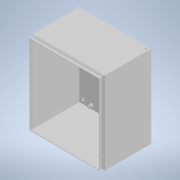
# Autodesk Inventor part: F161410HC1
Saved by Autodesk Inventor 2021 (Build 250183000, 183)
## iProperties
Created: 2025-08-10
Part Number: F161410HC1
Material: Generic
Catalog Web Link: www.cadenas.de
Description: JB CS Frame-JB
Vendor: RITTAL
Document SubType Name: Modeling
Designer: psAdmin
Manufacturer: RITTAL
Mass: 768.935 g
Surface Area: 10280.7 cm^2
Volume: 768.935 cm^3
Density: 1 g/cm^3
Appearance: PSOLRGB-175-175-175
Category: PARTsolutions
Company: RITTAL
Title: F161410HC1
Author: Cadenas PARTsolutions
Comments: JB
PSOL_IDENT_0: {$CADENAS_DATA/23d-libs/rittal/schaltschranksys/kleingeh/jb_parts/jb_frame.prj},178 {VTYP=3D},{NB=F1
PSOL_IDENT_1: 61410HC1},{LINA=F161410HC1},{NN=JB CS Frame},{DATE=20.08.2024 09:27:20},{GEOMDATE=07.07.2022 12:44:2
PSOL_IDENT_2: 1},{VERSION=},{LINEID=220},{WBVAR=DETAIL},{WBNUMERIC=DETAIL}  {NB=F161410HC1},{LINA=F161410HC1},{KT=
PSOL_IDENT_3: DUMMY},{PN=161410HC},{PNPLATE=JBMP1614},{WT=1.5000},{DETAIL=1},{WN=Y},{HM=400.00000},{BM=350.00000},
PSOL_IDENT_4: {TM=250.00000},{ST=224.03000},{ETFT=8.19000},{EPD=21.13000},{HHD=311.00000},{VHD=361.00000},{DMHD=28
PSOL_IDENT_5: 4.40000},{EW=0.00000},{EH=0.00000},{MPX=225.00000},{MPY=361.00000},{MPN=4},{NOH=2},{MAT=CS},{MT=cs}
NB: F161410HC1
NN: JB CS Frame
NT: JB
NBSYN: F$PN.$DETAIL.
LINA: F161410HC1
CATALOG: Rittal
PN: 161410HC
PNPLATE: JBMP1614
WT: 1.5
DETAIL: High
WN: Y
HM: 400
BM: 350
TM: 250
ST: 224.03
ETFT: 8.19
EPD: 21.13
HHD: 311
VHD: 361
DMHD: 284.4
EW: 0
EH: 0
MPX: 225
MPY: 361
MPN: 4
NOH: 2
MAT: CS
MT: cs
SUPPLIER: RITTAL
ARTICLENO: F161410HC1
BOMINFO: F161410HC1
CREATOR: CADENAS GmbH
Autodesk Inventor part; units mm, degrees
sketch "Sketch_1" plane through (0, 0, 0) normal (0, 0, 1) x (-1, 0, 0)
  line L0 (-175, -200) -> (175, -200)
  line L1 (175, -200) -> (175, 200)
  line L2 (175, 200) -> (-175, 200)
  line L3 (-175, 200) -> (-175, -200)
  constraints: 8 end point
extrude "Extrusion1" add sketch "Sketch_1" along normal blind 225.65
sketch "Sketch_2" plane through (0, 0, 1.5) normal (0, 0, 1) x (-1, 0, 0)
  line L0 (-173.5, -198.5) -> (173.5, -198.5)
  line L1 (173.5, -198.5) -> (173.5, 198.5)
  line L2 (173.5, 198.5) -> (-173.5, 198.5)
  line L3 (-173.5, 198.5) -> (-173.5, -198.5)
  constraints: 8 end point
extrude "Extrusion2" cut sketch "Sketch_2" along normal blind 225.65
sketch "Sketch_3" plane through (0, 0, 0) normal (-1, 0, 0) x (0, 0, -1)
  line L0 (-246.59, -193.8538) -> (-238.9625, -191.81)
  line L1 (-238.9625, -191.81) -> (-234.2713, -191.81)
  line L2 (-234.2713, -191.81) -> (-226.3742, -199.7071)
  arc A0 (-226.3742, -199.7071) -> (-225.6671, -200) centre (-225.6671, -199) ccw
  line L3 (-225.6671, -200) -> (-225.46, -200)
  line L4 (-225.46, -200) -> (-225.46, -198.5)
  line L5 (-225.46, -198.5) -> (-233.65, -190.31)
  line L6 (-233.65, -190.31) -> (-239.16, -190.31)
  line L7 (-239.16, -190.31) -> (-246.59, -192.3009)
  line L8 (-246.59, -192.3009) -> (-246.59, -193.8538)
  constraints: 18 end point, 2 point on circle, 1 centre point
extrude "Extrusion3" add sketch "Sketch_3" along normal mid plane 350
sketch "Sketch_4" plane through (0, 0, 0) normal (-1, 0, 0) x (0, 0, -1)
  line L0 (-246.59, 193.8538) -> (-246.59, 192.3009)
  line L1 (-246.59, 192.3009) -> (-239.16, 190.31)
  line L2 (-239.16, 190.31) -> (-233.65, 190.31)
  line L3 (-233.65, 190.31) -> (-225.46, 198.5)
  line L4 (-225.46, 198.5) -> (-225.46, 200)
  line L5 (-225.46, 200) -> (-225.6671, 200)
  arc A0 (-225.6671, 200) -> (-226.3742, 199.7071) centre (-225.6671, 199) ccw
  line L6 (-226.3742, 199.7071) -> (-234.2713, 191.81)
  line L7 (-234.2713, 191.81) -> (-238.9625, 191.81)
  line L8 (-238.9625, 191.81) -> (-246.59, 193.8538)
  constraints: 18 end point, 2 point on circle, 1 centre point
extrude "Extrusion4" add sketch "Sketch_4" along normal mid plane 350
sketch "Sketch_5" plane through (0, 0, 0) normal (0, -1, 0) x (-1, 0, 0)
  line L0 (-175, -225.65) -> (-166.81, -233.84)
  line L1 (-166.81, -233.84) -> (-166.81, -238.3425)
  line L2 (-166.81, -238.3425) -> (-169.0708, -246.78)
  line L3 (-169.0708, -246.78) -> (-167.5179, -246.78)
  line L4 (-167.5179, -246.78) -> (-165.31, -238.54)
  line L5 (-165.31, -238.54) -> (-165.31, -233.84)
  line L6 (-165.31, -233.84) -> (-173.5, -225.65)
  line L7 (-173.5, -225.65) -> (-175, -225.65)
  constraints: 16 end point
extrude "Extrusion5" add sketch "Sketch_5" along normal mid plane 400
sketch "Sketch_6" plane through (0, 0, 0) normal (0, -1, 0) x (-1, 0, 0)
  line L0 (165.31, -238.54) -> (167.5179, -246.78)
  line L1 (167.5179, -246.78) -> (169.0708, -246.78)
  line L2 (169.0708, -246.78) -> (166.81, -238.3425)
  line L3 (166.81, -238.3425) -> (166.81, -233.84)
  line L4 (166.81, -233.84) -> (175, -225.65)
  line L5 (175, -225.65) -> (173.5, -225.65)
  line L6 (173.5, -225.65) -> (165.31, -233.84)
  line L7 (165.31, -233.84) -> (165.31, -238.54)
  constraints: 16 end point
extrude "Extrusion6" add sketch "Sketch_6" along normal mid plane 400
sketch "Sketch_7" plane through (155, 0, 0) normal (-1, 0, 0) x (0, 0, -1)
  arc A0 (-3.5, -187.5) -> (-2, -189) centre (-2, -187.5) ccw
  line L0 (-2, -189) -> (0, -189)
  line L1 (0, -189) -> (0, -171)
  line L2 (0, -171) -> (-2, -171)
  arc A1 (-2, -171) -> (-3.5, -172.5) centre (-2, -172.5) ccw
  line L3 (-3.5, -172.5) -> (-3.5, -187.5)
  constraints: 8 end point, 4 point on circle, 2 centre point
extrude "Extrusion7" add sketch "Sketch_7" along normal mid plane 18
sketch "Sketch_8" plane through (-155, 0, 0) normal (-1, 0, 0) x (0, 0, -1)
  arc A0 (-3.5, -187.5) -> (-2, -189) centre (-2, -187.5) ccw
  line L0 (-2, -189) -> (0, -189)
  line L1 (0, -189) -> (0, -171)
  line L2 (0, -171) -> (-2, -171)
  arc A1 (-2, -171) -> (-3.5, -172.5) centre (-2, -172.5) ccw
  line L3 (-3.5, -172.5) -> (-3.5, -187.5)
  constraints: 8 end point, 4 point on circle, 2 centre point
extrude "Extrusion8" add sketch "Sketch_8" along normal mid plane 18
sketch "Sketch_9" plane through (155, 0, 0) normal (-1, 0, 0) x (0, 0, -1)
  arc A0 (-3.5, 172.5) -> (-2, 171) centre (-2, 172.5) ccw
  line L0 (-2, 171) -> (0, 171)
  line L1 (0, 171) -> (0, 189)
  line L2 (0, 189) -> (-2, 189)
  arc A1 (-2, 189) -> (-3.5, 187.5) centre (-2, 187.5) ccw
  line L3 (-3.5, 187.5) -> (-3.5, 172.5)
  constraints: 8 end point, 4 point on circle, 2 centre point
extrude "Extrusion9" add sketch "Sketch_9" along normal mid plane 18
sketch "Sketch_10" plane through (-155, 0, 0) normal (-1, 0, 0) x (0, 0, -1)
  arc A0 (-3.5, 172.5) -> (-2, 171) centre (-2, 172.5) ccw
  line L0 (-2, 171) -> (0, 171)
  line L1 (0, 171) -> (0, 189)
  line L2 (0, 189) -> (-2, 189)
  arc A1 (-2, 189) -> (-3.5, 187.5) centre (-2, 187.5) ccw
  line L3 (-3.5, 187.5) -> (-3.5, 172.5)
  constraints: 8 end point, 4 point on circle, 2 centre point
extrude "Extrusion10" add sketch "Sketch_10" along normal mid plane 18
sketch "Sketch_11" plane through (0, 180, 0) normal (0, -1, 0) x (-1, 0, 0)
  line L0 (-165, -1.5) -> (-165, -4.5)
  line L1 (-165, -4.5) -> (-145, -4.5)
  line L2 (-145, -4.5) -> (-145, -1.5)
  line L3 (-145, -1.5) -> (-146, -1.5)
  line L4 (-146, -1.5) -> (-146, -2)
  arc A0 (-147.5, -3.5) -> (-146, -2) centre (-147.5, -2) ccw
  line L5 (-147.5, -3.5) -> (-162.5, -3.5)
  arc A1 (-164, -2) -> (-162.5, -3.5) centre (-162.5, -2) ccw
  line L6 (-164, -2) -> (-164, -1.5)
  line L7 (-164, -1.5) -> (-165, -1.5)
  constraints: 16 end point, 4 point on circle, 2 centre point
extrude "Extrusion11" cut sketch "Sketch_11" along normal mid plane 18
sketch "Sketch_16" plane through (0, 180, 0) normal (0, -1, 0) x (-1, 0, 0)
  line L0 (145, -1.5) -> (145, -4.5)
  line L1 (145, -4.5) -> (165, -4.5)
  line L2 (165, -4.5) -> (165, -1.5)
  line L3 (165, -1.5) -> (164, -1.5)
  line L4 (164, -1.5) -> (164, -2)
  arc A0 (162.5, -3.5) -> (164, -2) centre (162.5, -2) ccw
  line L5 (162.5, -3.5) -> (147.5, -3.5)
  arc A1 (146, -2) -> (147.5, -3.5) centre (147.5, -2) ccw
  line L6 (146, -2) -> (146, -1.5)
  line L7 (146, -1.5) -> (145, -1.5)
  constraints: 16 end point, 4 point on circle, 2 centre point
extrude "Extrusion12" cut sketch "Sketch_16" along normal mid plane 18
sketch "Sketch_17" plane through (0, -180, 0) normal (0, -1, 0) x (-1, 0, 0)
  line L0 (-165, -1.5) -> (-165, -4.5)
  line L1 (-165, -4.5) -> (-145, -4.5)
  line L2 (-145, -4.5) -> (-145, -1.5)
  line L3 (-145, -1.5) -> (-146, -1.5)
  line L4 (-146, -1.5) -> (-146, -2)
  arc A0 (-147.5, -3.5) -> (-146, -2) centre (-147.5, -2) ccw
  line L5 (-147.5, -3.5) -> (-162.5, -3.5)
  arc A1 (-164, -2) -> (-162.5, -3.5) centre (-162.5, -2) ccw
  line L6 (-164, -2) -> (-164, -1.5)
  line L7 (-164, -1.5) -> (-165, -1.5)
  constraints: 16 end point, 4 point on circle, 2 centre point
extrude "Extrusion13" cut sketch "Sketch_17" along normal mid plane 18
sketch "Sketch_18" plane through (0, -180, 0) normal (0, -1, 0) x (-1, 0, 0)
  line L0 (145, -1.5) -> (145, -4.5)
  line L1 (145, -4.5) -> (165, -4.5)
  line L2 (165, -4.5) -> (165, -1.5)
  line L3 (165, -1.5) -> (164, -1.5)
  line L4 (164, -1.5) -> (164, -2)
  arc A0 (162.5, -3.5) -> (164, -2) centre (162.5, -2) ccw
  line L5 (162.5, -3.5) -> (147.5, -3.5)
  arc A1 (146, -2) -> (147.5, -3.5) centre (147.5, -2) ccw
  line L6 (146, -2) -> (146, -1.5)
  line L7 (146, -1.5) -> (145, -1.5)
  constraints: 16 end point, 4 point on circle, 2 centre point
extrude "Extrusion14" cut sketch "Sketch_18" along normal mid plane 18
sketch "Sketch_23" plane through (-155, 0, 0) normal (-1, 0, 0) x (0, 0, -1)
  arc A0 (-2, -188) -> (-0.5, -189.5) centre (-0.5, -188) ccw
  line L0 (-0.5, -189.5) -> (0, -189.5)
  line L1 (0, -189.5) -> (0, -171.5)
  line L2 (0, -171.5) -> (-0.5, -171.5)
  arc A1 (-0.5, -171.5) -> (-2, -173) centre (-0.5, -173) ccw
  line L3 (-2, -173) -> (-2, -188)
  constraints: 8 end point, 4 point on circle, 2 centre point
extrude "Extrusion15" cut sketch "Sketch_23" along normal mid plane 16
sketch "Sketch_24" plane through (-155, 0, 0) normal (-1, 0, 0) x (0, 0, -1)
  arc A0 (-2, 173) -> (-0.5, 171.5) centre (-0.5, 173) ccw
  line L0 (-0.5, 171.5) -> (0, 171.5)
  line L1 (0, 171.5) -> (0, 189.5)
  line L2 (0, 189.5) -> (-0.5, 189.5)
  arc A1 (-0.5, 189.5) -> (-2, 188) centre (-0.5, 188) ccw
  line L3 (-2, 188) -> (-2, 173)
  constraints: 8 end point, 4 point on circle, 2 centre point
extrude "Extrusion16" cut sketch "Sketch_24" along normal mid plane 16
sketch "Sketch_25" plane through (155, 0, 0) normal (-1, 0, 0) x (0, 0, -1)
  arc A0 (-2, 173) -> (-0.5, 171.5) centre (-0.5, 173) ccw
  line L0 (-0.5, 171.5) -> (0, 171.5)
  line L1 (0, 171.5) -> (0, 189.5)
  line L2 (0, 189.5) -> (-0.5, 189.5)
  arc A1 (-0.5, 189.5) -> (-2, 188) centre (-0.5, 188) ccw
  line L3 (-2, 188) -> (-2, 173)
  constraints: 8 end point, 4 point on circle, 2 centre point
extrude "Extrusion17" cut sketch "Sketch_25" along normal mid plane 16
sketch "Sketch_26" plane through (155, 0, 0) normal (-1, 0, 0) x (0, 0, -1)
  arc A0 (-2, -187.5) -> (-0.5, -189) centre (-0.5, -187.5) ccw
  line L0 (-0.5, -189) -> (0, -189)
  line L1 (0, -189) -> (0, -171)
  line L2 (0, -171) -> (-0.5, -171)
  arc A1 (-0.5, -171) -> (-2, -172.5) centre (-0.5, -172.5) ccw
  line L3 (-2, -172.5) -> (-2, -187.5)
  constraints: 8 end point, 4 point on circle, 2 centre point
extrude "Extrusion18" cut sketch "Sketch_26" along normal mid plane 16
sketch "Sketch_27" plane through (0, 0, 0) normal (0, 0, 1) x (-1, 0, 0)
  circle A0 centre (-155, -180) radius 4.35
  constraints: 1 centre point
extrude "Extrusion19" cut sketch "Sketch_27" along normal mid plane 8
sketch "Sketch_28" plane through (0, 0, 0) normal (0, 0, 1) x (-1, 0, 0)
  circle A0 centre (155, -180) radius 4.35
  constraints: 1 centre point
extrude "Extrusion20" cut sketch "Sketch_28" along normal mid plane 8
sketch "Sketch_29" plane through (0, 0, 0) normal (0, 0, 1) x (-1, 0, 0)
  circle A0 centre (-155, 180) radius 4.35
  constraints: 1 centre point
extrude "Extrusion21" cut sketch "Sketch_29" along normal mid plane 8
sketch "Sketch_30" plane through (0, 0, 0) normal (0, 0, 1) x (-1, 0, 0)
  circle A0 centre (155, 180) radius 4.35
  constraints: 1 centre point
extrude "Extrusion22" cut sketch "Sketch_30" along normal mid plane 8
sketch "Sketch_31" plane through (174.9829, -200, 225.6671) normal (0.7071, 0, 0.7071) x (-0.7071, 0, 0.7071)
  circle A0 centre (5.16, -57.8) radius 2.5
  constraints: 1 centre point
extrude "Extrusion23" cut sketch "Sketch_31" along normal mid plane 8
sketch "Sketch_32" plane through (174.9829, -200, 225.6671) normal (0.7071, 0, 0.7071) x (-0.7071, 0, 0.7071)
  circle A0 centre (5.16, -342.2) radius 2.5
  constraints: 1 centre point
extrude "Extrusion24" cut sketch "Sketch_32" along normal mid plane 8
sketch "Sketch_33" plane through (0, 0, 0) normal (-1, 0, 0) x (0, 0, -1)
  line L0 (-486.0789, 350) -> (-486.0789, -350)
  line L1 (-486.0789, -350) -> (-226.2713, -200)
  line L2 (-226.2713, -200) -> (-234.4613, -191.81)
  line L3 (-234.4613, -191.81) -> (-239.1525, -191.81)
  line L4 (-239.1525, -191.81) -> (-246.78, -193.8538)
  line L5 (-246.78, -193.8538) -> (-419.9851, -293.8538)
  line L6 (-419.9851, -293.8538) -> (-419.9851, 293.8538)
  line L7 (-419.9851, 293.8538) -> (-246.78, 193.8538)
  line L8 (-246.78, 193.8538) -> (-239.1525, 191.81)
  line L9 (-239.1525, 191.81) -> (-234.4613, 191.81)
  line L10 (-234.4613, 191.81) -> (-226.2713, 200)
  line L11 (-226.2713, 200) -> (-486.0789, 350)
  constraints: 24 end point
extrude "Extrusion25" cut sketch "Sketch_33" along normal mid plane 350
sketch "Sketch_34" plane through (0, 0, 0) normal (0, -1, 0) x (-1, 0, 0)
  line L0 (-325, -485.4576) -> (325, -485.4576)
  line L1 (325, -485.4576) -> (175, -225.65)
  line L2 (175, -225.65) -> (166.81, -233.84)
  line L3 (166.81, -233.84) -> (166.81, -238.3425)
  line L4 (166.81, -238.3425) -> (169.0708, -246.78)
  line L5 (169.0708, -246.78) -> (269.0708, -419.9851)
  line L6 (269.0708, -419.9851) -> (-269.0708, -419.9851)
  line L7 (-269.0708, -419.9851) -> (-169.0708, -246.78)
  line L8 (-169.0708, -246.78) -> (-166.81, -238.3425)
  line L9 (-166.81, -238.3425) -> (-166.81, -233.84)
  line L10 (-166.81, -233.84) -> (-175, -225.65)
  line L11 (-175, -225.65) -> (-325, -485.4576)
  constraints: 24 end point
extrude "Extrusion26" cut sketch "Sketch_34" along normal mid plane 400
sketch "Sketch_49" plane through (0, 0, 0) normal (-1, 0, 0) x (0, 0, -1)
  line L0 (-2.29, 210) -> (-2.29, 200)
  arc A0 (0, 197.71) -> (-2.29, 200) centre (-2.29, 197.71) ccw
  line L1 (0, 197.71) -> (0, -197.71)
  arc A1 (-2.29, -200) -> (0, -197.71) centre (-2.29, -197.71) ccw
  line L2 (-2.29, -200) -> (-2.29, -210)
  line L3 (-2.29, -210) -> (50, -210)
  line L4 (50, -210) -> (50, 210)
  line L5 (50, 210) -> (-2.29, 210)
  constraints: 12 end point, 4 point on circle, 2 centre point
extrude "Extrusion27" cut sketch "Sketch_49" along normal mid plane 350
sketch "Sketch_50" plane through (0, 0, 0) normal (0, -1, 0) x (-1, 0, 0)
  line L0 (-185, 50) -> (-185, -2.29)
  line L1 (-185, -2.29) -> (-175, -2.29)
  arc A0 (-172.71, 0) -> (-175, -2.29) centre (-172.71, -2.29) ccw
  line L2 (-172.71, 0) -> (172.71, 0)
  arc A1 (175, -2.29) -> (172.71, 0) centre (172.71, -2.29) ccw
  line L3 (175, -2.29) -> (185, -2.29)
  line L4 (185, -2.29) -> (185, 50)
  line L5 (185, 50) -> (-185, 50)
  constraints: 12 end point, 4 point on circle, 2 centre point
extrude "Extrusion28" cut sketch "Sketch_50" along normal mid plane 400
sketch "Sketch29" plane through (-173.4829, 200, 225.6671) normal (0, 1, 0) x (1, 0, 0)
  point P0 (335.7829, 211.8771)
hole "Hole1" at (162.3, 200, 13.79) direction (0, -1, 0) diameter 8.7 depth 4
sketch "Sketch_64" plane through (-112.5, 0, 0) normal (-1, 0, 0) x (0, 0, -1)
  line L0 (-1.5, 180.5) -> (-19.61, 180.5)
  line L1 (-19.61, 180.5) -> (-19.61, 183.88)
  arc A0 (-17.11, 186.38) -> (-19.61, 183.88) centre (-17.11, 183.88) ccw
  line L2 (-17.11, 186.38) -> (-16, 186.38)
  line L3 (-16, 186.38) -> (-16, 188.5)
  line L4 (-16, 188.5) -> (-14.5, 188.5)
  line L5 (-14.5, 188.5) -> (-14.5, 183.495)
  line L6 (-14.5, 183.495) -> (-12.5, 183.495)
  line L7 (-12.5, 183.495) -> (-12.5, 185.775)
  arc A1 (-10, 188.275) -> (-12.5, 185.775) centre (-10, 185.775) ccw
  line L8 (-10, 188.275) -> (-1.5, 188.275)
  line L9 (-1.5, 188.275) -> (-1.5, 186.45)
  line L10 (-1.5, 186.45) -> (-3, 186.45)
  arc A2 (-3, 186.45) -> (-5.5, 183.95) centre (-3, 183.95) ccw
  line L11 (-5.5, 183.95) -> (-5.5, 180.5)
  line L12 (-5.5, 180.5) -> (-19.61, 180.5)
  constraints: 26 end point, 6 point on circle, 3 centre point
revolve "Revolution1" add sketch "Sketch_64" angle 360 about axis through (-112.5, -180.5, 1.5) along (0, 0, -1)
sketch "Sketch_65" plane through (-112.5, 0, 0) normal (-1, 0, 0) x (0, 0, -1)
  line L0 (-1.5, -180.5) -> (-19.61, -180.5)
  line L1 (-19.61, -180.5) -> (-19.61, -177.12)
  arc A0 (-17.11, -174.62) -> (-19.61, -177.12) centre (-17.11, -177.12) ccw
  line L2 (-17.11, -174.62) -> (-16, -174.62)
  line L3 (-16, -174.62) -> (-16, -172.5)
  line L4 (-16, -172.5) -> (-14.5, -172.5)
  line L5 (-14.5, -172.5) -> (-14.5, -177.505)
  line L6 (-14.5, -177.505) -> (-12.5, -177.505)
  line L7 (-12.5, -177.505) -> (-12.5, -175.225)
  arc A1 (-10, -172.725) -> (-12.5, -175.225) centre (-10, -175.225) ccw
  line L8 (-10, -172.725) -> (-1.5, -172.725)
  line L9 (-1.5, -172.725) -> (-1.5, -174.55)
  line L10 (-1.5, -174.55) -> (-3, -174.55)
  arc A2 (-3, -174.55) -> (-5.5, -177.05) centre (-3, -177.05) ccw
  line L11 (-5.5, -177.05) -> (-5.5, -180.5)
  line L12 (-5.5, -180.5) -> (-19.61, -180.5)
  constraints: 26 end point, 6 point on circle, 3 centre point
revolve "Revolution2" add sketch "Sketch_65" angle 360 about axis through (-112.5, 180.5, 1.5) along (0, 0, -1)
sketch "Sketch_66" plane through (-112.5, -180.5, 19.61) normal (0, 0, 1) x (0, -1, 0)
  line L0 (-3, 0.8) -> (-3, -0.8)
  line L1 (-3, -0.8) -> (-0.8, -0.8)
  line L2 (-0.8, -0.8) -> (-0.8, -3)
  line L3 (-0.8, -3) -> (0.8, -3)
  line L4 (0.8, -3) -> (0.8, -0.8)
  line L5 (0.8, -0.8) -> (3, -0.8)
  line L6 (3, -0.8) -> (3, 0.8)
  line L7 (3, 0.8) -> (0.8, 0.8)
  line L8 (0.8, 0.8) -> (0.8, 3)
  line L9 (0.8, 3) -> (-0.8, 3)
  line L10 (-0.8, 3) -> (-0.8, 0.8)
  line L11 (-0.8, 0.8) -> (-3, 0.8)
  constraints: 24 end point
extrude "Extrusion29" cut sketch "Sketch_66" against normal blind 2.5
sketch "Sketch_67" plane through (-112.5, 180.5, 19.61) normal (0, 0, 1) x (0, -1, 0)
  line L0 (-3, 0.8) -> (-3, -0.8)
  line L1 (-3, -0.8) -> (-0.8, -0.8)
  line L2 (-0.8, -0.8) -> (-0.8, -3)
  line L3 (-0.8, -3) -> (0.8, -3)
  line L4 (0.8, -3) -> (0.8, -0.8)
  line L5 (0.8, -0.8) -> (3, -0.8)
  line L6 (3, -0.8) -> (3, 0.8)
  line L7 (3, 0.8) -> (0.8, 0.8)
  line L8 (0.8, 0.8) -> (0.8, 3)
  line L9 (0.8, 3) -> (-0.8, 3)
  line L10 (-0.8, 3) -> (-0.8, 0.8)
  line L11 (-0.8, 0.8) -> (-3, 0.8)
  constraints: 24 end point
extrude "Extrusion30" cut sketch "Sketch_67" against normal blind 2.5
sketch "Sketch_68" plane through (112.5, 0, 0) normal (-1, 0, 0) x (0, 0, -1)
  line L0 (-1.5, 180.5) -> (-19.61, 180.5)
  line L1 (-19.61, 180.5) -> (-19.61, 183.88)
  arc A0 (-17.11, 186.38) -> (-19.61, 183.88) centre (-17.11, 183.88) ccw
  line L2 (-17.11, 186.38) -> (-16, 186.38)
  line L3 (-16, 186.38) -> (-16, 188.5)
  line L4 (-16, 188.5) -> (-14.5, 188.5)
  line L5 (-14.5, 188.5) -> (-14.5, 183.495)
  line L6 (-14.5, 183.495) -> (-12.5, 183.495)
  line L7 (-12.5, 183.495) -> (-12.5, 185.775)
  arc A1 (-10, 188.275) -> (-12.5, 185.775) centre (-10, 185.775) ccw
  line L8 (-10, 188.275) -> (-1.5, 188.275)
  line L9 (-1.5, 188.275) -> (-1.5, 186.45)
  line L10 (-1.5, 186.45) -> (-3, 186.45)
  arc A2 (-3, 186.45) -> (-5.5, 183.95) centre (-3, 183.95) ccw
  line L11 (-5.5, 183.95) -> (-5.5, 180.5)
  line L12 (-5.5, 180.5) -> (-19.61, 180.5)
  constraints: 26 end point, 6 point on circle, 3 centre point
revolve "Revolution3" add sketch "Sketch_68" angle 360 about axis through (112.5, -180.5, 1.5) along (0, 0, -1)
sketch "Sketch_69" plane through (112.5, -180.5, 19.61) normal (0, 0, 1) x (0, -1, 0)
  line L0 (-3, 0.8) -> (-3, -0.8)
  line L1 (-3, -0.8) -> (-0.8, -0.8)
  line L2 (-0.8, -0.8) -> (-0.8, -3)
  line L3 (-0.8, -3) -> (0.8, -3)
  line L4 (0.8, -3) -> (0.8, -0.8)
  line L5 (0.8, -0.8) -> (3, -0.8)
  line L6 (3, -0.8) -> (3, 0.8)
  line L7 (3, 0.8) -> (0.8, 0.8)
  line L8 (0.8, 0.8) -> (0.8, 3)
  line L9 (0.8, 3) -> (-0.8, 3)
  line L10 (-0.8, 3) -> (-0.8, 0.8)
  line L11 (-0.8, 0.8) -> (-3, 0.8)
  constraints: 24 end point
extrude "Extrusion31" cut sketch "Sketch_69" against normal blind 2.5
sketch "Sketch_70" plane through (112.5, 0, 0) normal (-1, 0, 0) x (0, 0, -1)
  line L0 (-1.5, -180.5) -> (-19.61, -180.5)
  line L1 (-19.61, -180.5) -> (-19.61, -177.12)
  arc A0 (-17.11, -174.62) -> (-19.61, -177.12) centre (-17.11, -177.12) ccw
  line L2 (-17.11, -174.62) -> (-16, -174.62)
  line L3 (-16, -174.62) -> (-16, -172.5)
  line L4 (-16, -172.5) -> (-14.5, -172.5)
  line L5 (-14.5, -172.5) -> (-14.5, -177.505)
  line L6 (-14.5, -177.505) -> (-12.5, -177.505)
  line L7 (-12.5, -177.505) -> (-12.5, -175.225)
  arc A1 (-10, -172.725) -> (-12.5, -175.225) centre (-10, -175.225) ccw
  line L8 (-10, -172.725) -> (-1.5, -172.725)
  line L9 (-1.5, -172.725) -> (-1.5, -174.55)
  line L10 (-1.5, -174.55) -> (-3, -174.55)
  arc A2 (-3, -174.55) -> (-5.5, -177.05) centre (-3, -177.05) ccw
  line L11 (-5.5, -177.05) -> (-5.5, -180.5)
  line L12 (-5.5, -180.5) -> (-19.61, -180.5)
  constraints: 26 end point, 6 point on circle, 3 centre point
revolve "Revolution4" add sketch "Sketch_70" angle 360 about axis through (112.5, 180.5, 1.5) along (0, 0, -1)
sketch "Sketch_71" plane through (112.5, 180.5, 19.61) normal (0, 0, 1) x (0, -1, 0)
  line L0 (-3, 0.8) -> (-3, -0.8)
  line L1 (-3, -0.8) -> (-0.8, -0.8)
  line L2 (-0.8, -0.8) -> (-0.8, -3)
  line L3 (-0.8, -3) -> (0.8, -3)
  line L4 (0.8, -3) -> (0.8, -0.8)
  line L5 (0.8, -0.8) -> (3, -0.8)
  line L6 (3, -0.8) -> (3, 0.8)
  line L7 (3, 0.8) -> (0.8, 0.8)
  line L8 (0.8, 0.8) -> (0.8, 3)
  line L9 (0.8, 3) -> (-0.8, 3)
  line L10 (-0.8, 3) -> (-0.8, 0.8)
  line L11 (-0.8, 0.8) -> (-3, 0.8)
  constraints: 24 end point
extrude "Extrusion32" cut sketch "Sketch_71" against normal blind 2.5
ref_plane "dummy_XY" through (0, 200, 112.825) normal (0, 1, 0) x (-1, 0, 0)
ref_plane "dummy_YZ" through (0, 200, 112.825) normal (-1, 0, 0) x (0, 0, 1)
ref_plane "dummy_ZX" through (0, 200, 112.825) normal (0, 0, 1) x (0, 1, 0)
ref_plane "s1_XY" through (171.3342, 142.2, 229.3158) normal (0.7071, 0, 0.7071) x (-0.7071, 0, 0.7071)
ref_plane "s1_YZ" through (171.3342, 142.2, 229.3158) normal (-0.7071, 0, 0.7071) x (0, -1, 0)
ref_plane "s1_ZX" through (171.3342, 142.2, 229.3158) normal (0, -1, 0) x (0.7071, 0, 0.7071)
ref_plane "s2_XY" through (171.3342, -142.2, 229.3158) normal (0.7071, 0, 0.7071) x (-0.7071, 0, 0.7071)
ref_plane "s2_YZ" through (171.3342, -142.2, 229.3158) normal (-0.7071, 0, 0.7071) x (0, -1, 0)
ref_plane "s2_ZX" through (171.3342, -142.2, 229.3158) normal (0, -1, 0) x (0.7071, 0, 0.7071)
ref_plane "to_plate_XY" through (0, 0, 12.5) normal (0, 0, 1) x (-1, 0, 0)
ref_plane "to_plate_YZ" through (0, 0, 12.5) normal (-1, 0, 0) x (0, -1, 0)
ref_plane "to_plate_ZX" through (0, 0, 12.5) normal (0, -1, 0) x (0, 0, 1)
body "Solid1"
